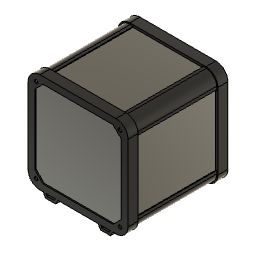
FrameBoxRoundEdge (Autodesk Fusion 360 design; units mm, degrees)
Autodesk Fusion 360 part; units mm, degrees
note: some values were not read from the file. Set by a fixed rule: which face or edge a step refers to.
sketch "masterSketch" plane through (0, 0, 0) normal (0, 1, 0) x (1, 0, 0)
  line L0 (-38, -50) -> (38, -50)
  line L1 (50, -38) -> (50, 38)
  line L2 (38, 50) -> (-38, 50)
  line L3 (-50, 38) -> (-50, -38)
  arc A0 (-50, -38) -> (-38, -50) centre (-38, -38) ccw
  arc A1 (-38, 50) -> (-50, 38) centre (-38, 38) ccw
  arc A2 (50, 38) -> (38, 50) centre (38, 38) ccw
  arc A3 (38, -50) -> (50, -38) centre (38, -38) ccw
  line L4 (47.6, -38) -> (47.6, 38)
  arc A4 (47.6, 38) -> (38, 47.6) centre (38, 38) ccw
  line L5 (38, 47.6) -> (-38, 47.6)
  arc A5 (-38, 47.6) -> (-47.6, 38) centre (-38, 38) ccw
  line L6 (-47.6, 38) -> (-47.6, -38)
  arc A6 (-47.6, -38) -> (-38, -47.6) centre (-38, -38) ccw
  line L7 (-38, -47.6) -> (38, -47.6)
  arc A7 (38, -47.6) -> (47.6, -38) centre (38, -38) ccw
  line L8 (48.8, -38) -> (48.8, 38)
  arc A8 (48.8, 38) -> (38, 48.8) centre (38, 38) ccw
  line L9 (38, 48.8) -> (-38, 48.8)
  arc A9 (-38, 48.8) -> (-48.8, 38) centre (-38, 38) ccw
  line L10 (-48.8, 38) -> (-48.8, -38)
  arc A10 (-48.8, -38) -> (-38, -48.8) centre (-38, -38) ccw
  line L11 (-38, -48.8) -> (38, -48.8)
  arc A11 (38, -48.8) -> (48.8, -38) centre (38, -38) ccw
  line L12 (48.4, -38) -> (48.4, 38)
  arc A12 (48.4, 38) -> (38, 48.4) centre (38, 38) ccw
  line L13 (38, 48.4) -> (-38, 48.4)
  arc A13 (-38, 48.4) -> (-48.4, 38) centre (-38, 38) ccw
  line L14 (-48.4, 38) -> (-48.4, -38)
  arc A14 (-48.4, -38) -> (-38, -48.4) centre (-38, -38) ccw
  line L15 (-38, -48.4) -> (38, -48.4)
  arc A15 (38, -48.4) -> (48.4, -38) centre (38, -38) ccw
  line L16 (-47.6, -38) -> (-44.8, -38)
  line L17 (-44.8, -38) -> (-44.8, -35)
  line L18 (-44.8, -35) -> (-43.2, -35)
  circle A16 centre (-42, -42) radius 2.25
  line L19 (-38, -47.6) -> (-38, -44.8)
  line L20 (-38, -44.8) -> (-35, -44.8)
  line L21 (-35, -44.8) -> (-35, -43.2)
  line L22 (-43.2, -35) -> (-35, -43.2)
  line L23 (-48.4, -35) -> (-47.6, -35)
  line L24 (-35, -47.6) -> (-35, -48.4)
  line L25 (0, -1.75) -> (0, -22.5)
  line L26 (44.8, -35) -> (43.2, -35)
  line L27 (43.2, -35) -> (35, -43.2)
  line L28 (35, -44.8) -> (35, -43.2)
  line L29 (38, -44.8) -> (35, -44.8)
  line L30 (38, -47.6) -> (38, -44.8)
  line L31 (35, -47.6) -> (35, -48.4)
  line L32 (48.4, -35) -> (47.6, -35)
  circle A17 centre (42, -42) radius 2.25
  line L33 (44.8, -38) -> (44.8, -35)
  line L34 (47.6, -38) -> (44.8, -38)
  line L35 (1.75, 0) -> (22.5, 0)
  line L36 (-47.6, 38) -> (-44.8, 38)
  line L37 (-44.8, 38) -> (-44.8, 35)
  line L38 (-44.8, 35) -> (-43.2, 35)
  line L39 (-43.2, 35) -> (-35, 43.2)
  line L40 (-35, 44.8) -> (-35, 43.2)
  line L41 (-38, 44.8) -> (-35, 44.8)
  line L42 (-38, 47.6) -> (-38, 44.8)
  line L43 (-35, 47.6) -> (-35, 48.4)
  line L44 (-48.4, 35) -> (-47.6, 35)
  circle A18 centre (-42, 42) radius 2.25
  line L45 (35, 47.6) -> (35, 48.4)
  line L46 (38, 47.6) -> (38, 44.8)
  line L47 (38, 44.8) -> (35, 44.8)
  line L48 (35, 44.8) -> (35, 43.2)
  line L49 (43.2, 35) -> (35, 43.2)
  line L50 (44.8, 35) -> (43.2, 35)
  line L51 (44.8, 38) -> (44.8, 35)
  line L52 (47.6, 38) -> (44.8, 38)
  line L53 (48.4, 35) -> (47.6, 35)
  circle A19 centre (42, 42) radius 2.25
  line L54 (-35, -43.2) -> (35, -43.2)
  line L55 (43.2, -35) -> (43.2, 35)
  line L56 (35, 43.2) -> (-35, 43.2)
  line L57 (-43.2, 35) -> (-43.2, -35)
  line L58 (-35, -48.4) -> (-35, -48.8)
  line L59 (-48.4, -35) -> (-48.8, -35)
  line L60 (35, -48.4) -> (35, -48.8)
  line L61 (48.4, -35) -> (48.8, -35)
  line L62 (-48.4, 35) -> (-48.8, 35)
  line L63 (-35, 48.4) -> (-35, 48.8)
  line L64 (35, 48.4) -> (35, 48.8)
  line L65 (48.4, 35) -> (48.8, 35)
  line L66 (-35, 50) -> (-32.5, 54.3301)
  line L67 (-35, 50) -> (-31, 50) construction
  line L68 (-32.5, 54.3301) -> (-22.5, 54.3301)
  line L69 (-22.5, 54.3301) -> (-20, 50)
  line L70 (-22.5, 54.3301) -> (-22, 54.3301) construction
  line L71 (-32.9215, 48.8) -> (-31.1144, 51.9301)
  line L72 (-31.1144, 51.9301) -> (-23.8856, 51.9301)
  line L73 (-23.8856, 51.9301) -> (-22.0785, 48.8)
  line L74 (35, 50) -> (32.5, 54.3301)
  line L75 (32.5, 54.3301) -> (22.5, 54.3301)
  line L76 (22.5, 54.3301) -> (20, 50)
  line L77 (23.8856, 51.9301) -> (22.0785, 48.8)
  line L78 (31.1144, 51.9301) -> (23.8856, 51.9301)
  line L79 (32.9215, 48.8) -> (31.1144, 51.9301)
  circle A20 centre (-42, -42) radius 1.75
  circle A21 centre (42, -42) radius 1.75
  circle A22 centre (-42, 42) radius 1.75
  circle A23 centre (42, 42) radius 1.75
  dimension "d10" = 50
  dimension "d11" = 50
  dimension "d12" = 100
  dimension "d13" = 100
  dimension "d14" = 12
  dimension "d19" = 2.8
  dimension "d20" = 1.6
  dimension "d21" = 4.5
  dimension "d22" = 2.8
  dimension "d23" = 1.6
  dimension "d25" = 3
  dimension "d26" = 3
  dimension "d27" = 2.8
  dimension "d28" = 2.8
  dimension "d65" = 5
  dimension "d66" = 60
  dimension "d67" = 10
  dimension "d68" = 60
  dimension "d69" = 2.4
  dimension "d72" = 70
  dimension "d73" = 70
  dimension "d102" = 3.5
  constraint horizontal L0
  constraint vertical L1
  constraint horizontal L2
  constraint vertical L3
  constraint tangent L0 A0
  constraint tangent L3 A0
  constraint tangent L2 A1
  constraint tangent L3 A1
  constraint equal A0 A1
  constraint tangent L1 A2
  constraint tangent L2 A2
  constraint equal A0 A2
  constraint tangent L0 A3
  constraint tangent L1 A3
  constraint equal A0 A3
  constraint perpendicular L6 L16
  constraint perpendicular L16 L17
  constraint perpendicular L17 L18
  constraint perpendicular L7 L19
  constraint perpendicular L19 L20
  constraint perpendicular L20 L21
  constraint coincident L14 L23.start
  constraint coincident L6 L23.end
  constraint perpendicular L6 L23
  constraint coincident L7 L24.start
  constraint coincident L15 L24.end
  constraint perpendicular L15 L24
  constraint collinear L21 L24
  constraint collinear L18 L23
  constraint symmetric L6.end L25 L4.start
  constraint symmetric A6.end L25 L7.end
  constraint symmetric L16.end L25 L33.start
  constraint symmetric L17.end L25 L26.start
  constraint symmetric L18.end L25 L26.end
  constraint symmetric A16 L25 A17
  constraint symmetric L19.end L25 L29.start
  constraint symmetric L20.end L25 L28.start
  constraint symmetric L21.end L25 L27.end
  constraint symmetric L23.start L25 L32.start
  constraint symmetric L23.end L25 L32.end
  constraint symmetric L24.start L25 L31.start
  constraint symmetric L24.end L25 L31.end
  constraint symmetric L6.end L35 A5.end
  constraint symmetric A6.end L35 L5.end
  constraint symmetric L16.end L35 L36.end
  constraint symmetric L17.end L35 L37.end
  constraint symmetric L18.end L35 L38.end
  constraint symmetric A16 L35 A18
  constraint symmetric L19.end L35 L41.start
  constraint symmetric L20.end L35 L40.start
  constraint symmetric L21.end L35 L39.end
  constraint symmetric L23.start L35 L44.start
  constraint symmetric L23.end L35 L44.end
  constraint symmetric L24.start L35 L43.start
  constraint symmetric L24.end L35 L43.end
  constraint symmetric L26.start L35 L50.start
  constraint symmetric L26.end L35 L49.start
  constraint symmetric L27.end L35 L48.end
  constraint symmetric L28.start L35 L47.end
  constraint symmetric L29.start L35 L46.end
  constraint symmetric L7.end L35 A4.end
  constraint symmetric L31.start L35 L45.start
  constraint symmetric L31.end L35 L45.end
  constraint symmetric L32.start L35 L53.start
  constraint symmetric L32.end L35 L53.end
  constraint symmetric A17 L35 A19
  constraint symmetric L33.start L35 L51.start
  constraint symmetric L4.start L35 L4.end
  constraint coincident L11 L58.end
  constraint perpendicular L11 L58
  constraint coincident L10 L59.end
  constraint perpendicular L10 L59
  constraint symmetric L25 L58.end L60.end
  constraint symmetric L25 L59.end L61.end
  constraint symmetric L35 L58.end L63.end
  constraint symmetric L35 L59.end L62.end
  constraint symmetric L35 L31.end L45.end
  constraint symmetric L35 L60.end L64.end
  constraint symmetric L35 L32.start L53.start
  constraint symmetric L35 L61.end L65.end
  constraint horizontal L67
  constraint coincident L2 L66.start
  constraint horizontal L68
  constraint horizontal L70
  constraint coincident L2 L69.end
  constraint symmetric L25 L66.start L74.start
  constraint symmetric L25 L66.end L74.end
  constraint symmetric L25 L68.end L75.end
  constraint symmetric L25 L69.end L76.end
  constraint symmetric L25 L71.start L79.start
  constraint symmetric L25 L71.end L78.start
  constraint symmetric L25 L72.end L77.start
  constraint symmetric L25 L73.end L77.end
  constraint vertical L43.end L66.start
  constraint concentric A16 A20
  constraint symmetric L25 A20 A21
  constraint symmetric L35 A20 A22
  constraint symmetric L35 A21 A23
  measures "d10" distance of origin L0
  measures "d11" distance of origin L3
  measures "d12" distance of L1 L3
  measures "d13" distance of L0 L2
  measures "d14" radius of A0
  measures "d19" distance of L6.end L16.end
  measures "d20" distance of L17.end L18.end
  measures "d21" diameter of A16
  measures "d22" distance of A6.end L19.end
  measures "d23" distance of L20.end L21.end
  measures "d25" distance of L19 L24
  measures "d26" distance of L16 L23
  measures "d27" distance of L17 A16.centre
  measures "d28" distance of A16.centre L20
  measures "d65" distance of L66.start L66.end
  measures "d66" angle of L66 L67
  measures "d67" distance of L66.end L68.end
  measures "d68" angle of L69 L70
  measures "d72" distance of L21.end L27.end
  measures "d73" distance of L18.end L38.end
  measures "d102" diameter of A20
extrude "Extrude1" add sketch "masterSketch" along normal blind 10 contours L0 L1 L2 L3 A0 A1 A2 A3 L8 A8 L9 A9 L10 A10 L11 A11 L71 L79 | L2 L66 L68 L69 L71 L72 L73 | L2 L74 L75 L76 L77 L78 L79 | L2 L9 L71 L73 | L2 L9 L77 L79 | L2 L9 L73 L77 | L9 L13 L63 L64 | L5 L13 L43 L45 | L10 L14 L59 L62 | L8 L12 L61 L65 | L6 L14 L23 L44 | L4 L12 L32 L53 | L11 L15 L58 L60 | L7 L15 L24 L31 makes body 1 in component "faceFrame"
extrude "Extrude2" add sketch "masterSketch" along normal blind 1.2 contours L9 A9 L10 L13 A13 L14 L62 L63 | L8 A8 L9 L12 A12 L13 L64 L65 | L5 A5 L6 L13 A13 L14 L43 L44 | L4 A4 L5 L12 A12 L13 L45 L53 | L5 L40 L41 L42 L46 L47 L48 L56 | A5 L36 L37 L38 L39 L40 L41 L42 | A4 L46 L47 L48 L49 L50 L51 L52 | L10 A10 L11 L14 A14 L15 L58 L59 | L6 L16 L17 L18 L36 L37 L38 L57 | L8 L11 A11 L12 L15 A15 L60 L61 | L4 L26 L33 L34 L50 L51 L52 L55 | L6 A6 L7 L14 A14 L15 L23 L24 | L4 L7 A7 L12 L15 A15 L31 L32 | A6 L16 L17 L18 L19 L20 L21 L22 | A7 L26 L27 L28 L29 L30 L33 L34 | L7 L19 L20 L21 L28 L29 L30 L54 | A16 | A17 | A18 | A19 bodies 1 in component "faceFrame"
extrude "Extrude1'" add sketch "masterSketch" along normal blind 92.8 separate body contours L5 A5 L6 L13 A13 L14 L43 L44 | L4 A4 L5 L12 A12 L13 L45 L53 | A5 L36 L37 L38 L39 L40 L41 L42 | A4 L46 L47 L48 L49 L50 L51 L52 | L6 A6 L7 L14 A14 L15 L23 L24 | L4 L7 A7 L12 L15 A15 L31 L32 | A6 L16 L17 L18 L19 L20 L21 L22 | A7 L26 L27 L28 L29 L30 L33 L34 makes body 2 at (-42.7656, 61.8667, 47.2439) makes body 3 at (48.3882, 61.8667, 38.4949) makes body 4 at (45.5268, 61.8667, -45.1768) makes body 5 at (-47.2439, 61.8667, -42.7656) in component "rail1"
move_face "OffsetFaces1" offset -0.4 8 faces at (35, 4.1333, 48) (48.4, 4.1333, 35) (-35, 4.1333, 48) (-48, 4.1333, 35) (-35, 4.1333, -48) (-48.4, 4.1333, -35) (48, 4.1333, -35) (35, 4.1333, -48) on bodies 1 in component "faceFrame"
extrude "Extrude1''" add sketch "masterSketch" along normal blind 2.4 separate body contours L5 L40 L41 L42 L46 L47 L48 L56 | A5 L36 L37 L38 L39 L40 L41 L42 | A4 L46 L47 L48 L49 L50 L51 L52 | L6 L16 L17 L18 L36 L37 L38 L57 | L4 L26 L33 L34 L50 L51 L52 L55 | L22 L27 L39 L49 L54 L55 L56 L57 | A6 L16 L17 L18 L19 L20 L21 L22 | A7 L26 L27 L28 L29 L30 L33 L34 | L7 L19 L20 L21 L28 L29 L30 L54 | A16 | A17 | A18 | A19 makes body 6 in component "front"
sketch "Sketch1" plane through (0, 0, 0) normal (0, 0, 1) x (1, 0, 0) in component "top"
  line L0 (-37.6, 95.6) -> (37.6, 95.6)
  line L1 (37.6, 95.6) -> (37.6, 3.6)
  line L2 (37.6, 3.6) -> (-37.6, 3.6)
  line L3 (-37.6, 3.6) -> (-37.6, 95.6)
  line L4 (0, 1.75) -> (0, 22.5)
  dimension "d71" = 92
  dimension "d74" = 75.2
  dimension "d75" = 37.6
  dimension "d76" = 3.6
  constraint horizontal L0
  constraint vertical L1
  constraint horizontal L2
  constraint vertical L3
  measures "d71" distance of L0 L2
  measures "d74" distance of L1 L3
  measures "d75" distance of L3 L4
  measures "d76" distance of origin L2
extrude "Extrude1'''" add sketch "Sketch1" along normal blind 2.4 separate body makes body 7 in component "top"
chamfer "Chamfer1" distance 0.8 angle 45 12 edges at (-37.6, 49.6, 0) (0, 3.6, 0) (37.6, 49.6, 0) (0, 95.6, 0) (-37.6, 49.6, 2.4) (0, 95.6, 2.4) (0, 3.6, 2.4) (37.6, 49.6, 2.4) (37.6, 3.6, 1.2) (37.6, 95.6, 1.2) (-37.6, 95.6, 1.2) (-37.6, 3.6, 1.2) on bodies 7 in component "top"
sketch "Sketch1 (2)" plane through (0, 0, 0) normal (1, 0, 0) x (0, 0, -1) in component "right"
  line L0 (-31.5949, 96.3432) -> (43.6051, 96.3432)
  line L1 (43.6051, 96.3432) -> (43.6051, 4.3432)
  line L2 (43.6051, 4.3432) -> (-31.5949, 4.3432)
  line L3 (-31.5949, 4.3432) -> (-31.5949, 96.3432)
  dimension "d88" = 92
  dimension "d89" = 75.2
  constraint horizontal L0
  constraint vertical L1
  constraint horizontal L2
  constraint vertical L3
  measures "d88" distance of L0 L2
  measures "d89" distance of L1 L3
extrude "Extrude1''''" add sketch "Sketch1 (2)" along normal blind 2.4 separate body makes body 8 in component "right"
chamfer "Chamfer1'" distance 0.8 angle 45 12 edges at (2.4, 50.3432, 31.5949) (2.4, 96.3432, -6.0051) (2.4, 50.3432, -43.6051) (0, 50.3432, 31.5949) (0, 96.3432, -6.0051) (0, 50.3432, -43.6051) (1.2, 4.3432, 31.5949) (1.2, 4.3432, -43.6051) (1.2, 96.3432, -43.6051) (1.2, 96.3432, 31.5949) (0, 4.3432, -6.0051) (2.4, 4.3432, -6.0051) on bodies 8 in component "right"
move_face "OffsetFaces1'" offset -0.4 16 faces at (-37, 0.8, 47.6) (11.6667, 1.6, 47.6) (37, 1.6, 47.6) (-45.5461, 1.6, 43.9343) (-47.6, 0.8, -37) (-47.6, 1.6, 11.6667) (-47.6, 0.8, 36) (-43.9343, 1.6, -45.5461) (-11.6667, 1.6, -47.6) (-36, 0.8, -47.6) (37, 0.8, -47.6) (42.8, 1.6, -46.3138) (47.6, 0.8, 37) (47.6, 0.8, -11.6667) (47.6, 0.8, -36) (45.5461, 1.6, 43.9343) on bodies 6 in component "front"
sketch "Sketch1 (3)" plane through (0, 0, 0) normal (0, 0, 1) x (1, 0, 0) in component "bottom"
  line L0 (-37.6, 95.6) -> (37.6, 95.6)
  line L1 (37.6, 95.6) -> (37.6, 3.6)
  line L2 (37.6, 3.6) -> (-37.6, 3.6)
  line L3 (-37.6, 3.6) -> (-37.6, 95.6)
  line L4 (0, 1.75) -> (0, 22.5)
  dimension "d71_1" = 92
  dimension "d74_1" = 75.2
  dimension "d75_1" = 37.6
  dimension "d76_1" = 3.6
  constraint horizontal L0
  constraint vertical L1
  constraint horizontal L2
  constraint vertical L3
  measures "d71_1" distance of L0 L2
  measures "d74_1" distance of L1 L3
  measures "d75_1" distance of L3 L4
  measures "d76_1" distance of origin L2
extrude "Extrude1'''''" add sketch "Sketch1 (3)" along normal blind 2.4 separate body makes body 9 in component "bottom"
chamfer "Chamfer1''" distance 0.8 angle 45 12 edges at (-37.6, 49.6, 0) (0, 3.6, 0) (37.6, 49.6, 0) (0, 95.6, 0) (-37.6, 49.6, 2.4) (0, 95.6, 2.4) (0, 3.6, 2.4) (37.6, 49.6, 2.4) (37.6, 3.6, 1.2) (37.6, 95.6, 1.2) (-37.6, 95.6, 1.2) (-37.6, 3.6, 1.2) on bodies 9 in component "bottom"
sketch "Sketch1 (4)" plane through (0, 0, 0) normal (1, 0, 0) x (0, 0, -1) in component "left"
  line L0 (-31.5949, 96.3432) -> (43.6051, 96.3432)
  line L1 (43.6051, 96.3432) -> (43.6051, 4.3432)
  line L2 (43.6051, 4.3432) -> (-31.5949, 4.3432)
  line L3 (-31.5949, 4.3432) -> (-31.5949, 96.3432)
  dimension "d88_1" = 92
  dimension "d89_1" = 75.2
  constraint horizontal L0
  constraint vertical L1
  constraint horizontal L2
  constraint vertical L3
  measures "d88_1" distance of L0 L2
  measures "d89_1" distance of L1 L3
extrude "Extrude1''''''" add sketch "Sketch1 (4)" along normal blind 2.4 separate body makes body 10 in component "left"
chamfer "Chamfer1'''" distance 0.8 angle 45 12 edges at (2.4, 50.3432, 31.5949) (2.4, 96.3432, -6.0051) (2.4, 50.3432, -43.6051) (0, 50.3432, 31.5949) (0, 96.3432, -6.0051) (0, 50.3432, -43.6051) (1.2, 4.3432, 31.5949) (1.2, 4.3432, -43.6051) (1.2, 96.3432, -43.6051) (1.2, 96.3432, 31.5949) (0, 4.3432, -6.0051) (2.4, 4.3432, -6.0051) on bodies 10 in component "left"
extrude "Extrude1'''''''" add sketch "masterSketch" along normal blind 2.4 separate body contours L5 L40 L41 L42 L46 L47 L48 L56 | A5 L36 L37 L38 L39 L40 L41 L42 | A4 L46 L47 L48 L49 L50 L51 L52 | L6 L16 L17 L18 L36 L37 L38 L57 | L4 L26 L33 L34 L50 L51 L52 L55 | L22 L27 L39 L49 L54 L55 L56 L57 | A6 L16 L17 L18 L19 L20 L21 L22 | A7 L26 L27 L28 L29 L30 L33 L34 | L7 L19 L20 L21 L28 L29 L30 L54 | A16 | A17 | A18 | A19 makes body 11 in component "back"
move_face "OffsetFaces1''" offset -0.4 16 faces at (-37, 0.8, 47.6) (11.6667, 1.6, 47.6) (37, 1.6, 47.6) (-45.5461, 1.6, 43.9343) (-47.6, 0.8, -37) (-47.6, 1.6, 11.6667) (-47.6, 0.8, 36) (-43.9343, 1.6, -45.5461) (-11.6667, 1.6, -47.6) (-36, 0.8, -47.6) (37, 0.8, -47.6) (42.8, 1.6, -46.3138) (47.6, 0.8, 37) (47.6, 0.8, -11.6667) (47.6, 0.8, -36) (45.5461, 1.6, 43.9343) on bodies 11 in component "back"
component "faceFrame" placed x (1, 0, 0) y (0, 1, 0) z (0, 0, 1) at (0, 0, 0)
component "rail1" placed x (1, 0, 0) y (0, 1, 0) z (0, 0, 1) at (0, 3.6, 0)
component "front" placed x (1, 0, 0) y (0, 1, 0) z (0, 0, 1) at (0, 1.2, 0)
component "faceFrame" placed x (-1, 0, 0) y (0, -1, 0) z (0, 0, 1) at (0, 100, 0)
component "top" placed x (1, 0, 0) y (0, 1, 0) z (0, 0, 1) at (0, 0.4, 45)
component "right" placed x (1, 0, 0) y (0, 1, 0) z (0, 0, 1) at (45, -0.3432, 6.0051)
component "bottom" placed x (1, 0, 0) y (0, 1, 0) z (0, 0, 1) at (0, 0.4, -47.4)
component "left" placed x (1, 0, 0) y (0, 1, 0) z (0, 0, 1) at (-47.4, -0.3432, 6.4051)
component "back" placed x (-1, 0, 0) y (0, -1, 0) z (0, 0, 1) at (0, 98.8, 0)
equation "boxWidth = 100 mm"
equation "boxHeight = 100 mm"
equation "boxDepth = 100 mm"
equation "frameThickness = 2.4 mm"
equation "frameClearance = 0.4 mm"
equation "sideThickness = 2.4 mm"
equation "sideClearance = 0.4 mm"
equation "d10 = boxHeight / 2"
equation "d11 = boxWidth / 2"
equation "d12 = boxWidth"
equation "d13 = boxHeight"
equation "d15 = -frameThickness"
equation "d16 = -( frameThickness - railThickness - frameClearance )"
equation "railThickness = 0.8 mm"
equation "d18 = -( frameThickness - railThickness )"
equation "d19 = sideThickness + sideClearance"
equation "d20 = 2 * railThickness"
equation "d23 = 2 * railThickness"
equation "d37 = frameFrontFacingThickness"
equation "d39 = boxDepth - ( 2 * frameFrontFacingThickness ) - ( 2 * sideThickness )"
equation "d41 = -frameClearance"
equation "d42 = sideThickness"
equation "frameFrontFacingThickness = 1.2 mm"
equation "d71 = boxDepth - ( 2 * frameFrontFacingThickness ) - ( 2 * frameThickness ) - ( 2 * frameClearance )"
equation "d74 = d72 + 2 * ( 3 mm - frameClearance )"
equation "d75 = d74 / 2"
equation "d76 = frameFrontFacingThickness + frameThickness"
equation "d77 = sideThickness"
equation "d81 = sideClearance"
equation "d82 = -3 * frameClearance"
equation "d88 = boxDepth - ( 2 * frameFrontFacingThickness ) - ( 2 * frameThickness ) - ( 2 * sideClearance )"
equation "d89 = d73 + 2 * ( 3 mm - sideClearance )"
equation "d90 = sideThickness"
equation "d94 = -frameClearance"
equation "d95 = 3 * sideClearance"
equation "d101 = -sideClearance"
equation "d71_1 = boxDepth - ( 2 * frameFrontFacingThickness ) - ( 2 * frameThickness ) - ( 2 * frameClearance )"
equation "d74_1 = d72 + 2 * ( 3 mm - frameClearance )"
equation "d75_1 = d74_1 / 2"
equation "d76_1 = frameFrontFacingThickness + frameThickness"
equation "d77_1 = sideThickness"
equation "d88_1 = boxDepth - ( 2 * frameFrontFacingThickness ) - ( 2 * frameThickness ) - ( 2 * sideClearance )"
equation "d89_1 = d73 + 2 * ( 3 mm - sideClearance )"
equation "d90_1 = sideThickness"
equation "d42_1 = sideThickness"
equation "d101_1 = -sideClearance"
equation "d116 = -sideClearance"
equation "d117 = sideClearance * 3"
equation "d121 = -sideClearance * 3"
named bodies: "rail1", "rail2", "rail3", "rail4", "face1"
